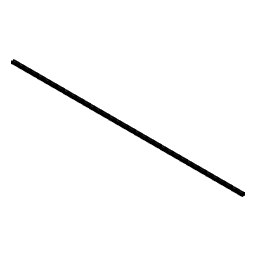
Aluminium U-channel X v1 (Autodesk Fusion 360 design; units mm, degrees)
Autodesk Fusion 360 part; units mm, degrees
sketch "Sketch1" plane through (0, 0, 0) normal (1, 0, 0) x (0, 1, 0)
  line L0 (-8, 0) -> (8, 0)
  line L1 (8, 0) -> (8, 12)
  line L2 (8, 12) -> (6, 12)
  line L3 (-8, 0) -> (-8, 12)
  line L4 (-8, 12) -> (-6, 12)
  line L5 (6, 12) -> (6, 2)
  line L6 (6, 2) -> (-6, 2)
  line L7 (-6, 2) -> (-6, 12)
  dimension "d26" = 16
  dimension "d27" = 12
  dimension "d28" = 2
  dimension "d29" = 12
  dimension "d30" = 2
  dimension "d31" = 10
  dimension "d32" = 12
  dimension "d33" = 10
  constraint perpendicular L0 L1
  constraint perpendicular L0 L3
  constraint perpendicular L3 L4
  constraint midpoint origin L0
  constraint perpendicular L2 L5
  constraint perpendicular L5 L6
  constraint perpendicular L4 L7
  measures "d26" distance of L0.start L0.end
  measures "d27" distance of L0.end L1.end
  measures "d28" distance of L1.end L2.end
  measures "d29" distance of L0.start L3.end
  measures "d30" distance of L3.end L4.end
  measures "d31" distance of L2.end L5.end
  measures "d32" distance of L5.end L6.end
  measures "d33" distance of L6.end L4.end
sketch "Sketch2" plane through (0, 0, 1.3) normal (0, 0, 1) x (-1, 0, 0)
  line L0 (800, 3) -> (-800, 3)
  line L1 (-800, 3) -> (-800, -3)
  line L2 (-800, -3) -> (800, -3)
  line L3 (800, -3) -> (800, 3)
  line L4 (800, 0) -> (792, 0) construction
  circle A0 centre (792, 0) radius 2
  line L5 (792, 0) -> (750, 0) construction
  circle A1 centre (750, 0) radius 2
  line L6 (-800, 0) -> (-792, 0) construction
  circle A2 centre (-792, 0) radius 2
  line L7 (-792, 0) -> (-750, 0) construction
  circle A3 centre (-750, 0) radius 2
  dimension "d14" = 8
  dimension "d15" = 4
  dimension "d16" = 42
  dimension "d17" = 4
  dimension "d18" = 8
  dimension "d19" = 4
  dimension "d20" = 42
  dimension "d21" = 4
  constraint midpoint L3 L4.start
  constraint perpendicular L3 L4
  constraint coincident L4.end A0.centre
  constraint parallel L4 L5
  constraint coincident L5.end A1.centre
  constraint midpoint L1 L6.start
  constraint perpendicular L1 L6
  constraint coincident L6.end A2.centre
  constraint parallel L6 L7
  constraint coincident L7.end A3.centre
  measures "d14" distance of L4.start L4.end
  measures "d15" diameter of A0
  measures "d16" distance of L4.end L5.end
  measures "d17" diameter of A1
  measures "d18" distance of L6.start L6.end
  measures "d19" diameter of A2
  measures "d20" distance of L6.end L7.end
  measures "d21" diameter of A3
extrude "Extrude3" add sketch "Sketch1" along normal mid plane 1600
extrude "Extrude4" cut sketch "Sketch2" along normal blind 0.7 and the other way blind 1.3 contours A0 | A1 | A2 | A3
